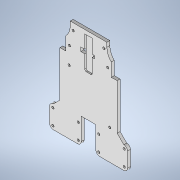
# Autodesk Inventor part: Основа робота
Saved by Autodesk Inventor 2020 (Build 240168000, 168)
## iProperties
Created: 2021-02-28
Part Number: Основа робота
Material: Типовые
Document SubType Name: Обычные детали
Designer: Антон
Density: 1 g/cm^3
Appearance: По умолчанию
Mass: 52.0111 g
Surface Area: 352.197 cm^2
Volume: 52.0111 cm^3
Sheet Metal Rule: По умолчанию
Author: Антон
Autodesk Inventor part; units mm, degrees
ref_plane "YZ Plane" through (0, 0, 0) normal (1, 0, 0) x (0, 1, 0)
ref_plane "XZ Plane" through (0, 0, 0) normal (0, 1, 0) x (-1, 0, 0)
ref_plane "XY Plane" through (0, 0, 0) normal (0, 0, 1) x (1, 0, 0)
sketch "Эскиз1" plane through (0, 0, 0) normal (0, 0, 1) x (1, 0, 0)
  line L0 (0, 0) -> (39, 0)
  line L1 (39, 0) -> (39, 139.6)
  line L2 (39, 139.6) -> (0, 139.6)
  line L3 (0, 139.6) -> (0, 0)
  line L4 (0, 0) -> (-14.05, 0)
  line L5 (-14.05, 0) -> (-14.05, 30.3)
  line L6 (-14.05, 30.3) -> (0, 30.3)
  line L7 (0, 30.3) -> (0, 0)
  line L8 (-14.05, 0) -> (-9.5, 0)
  line L9 (-9.5, 0) -> (-9.5, 4.55)
  line L10 (-9.5, 4.55) -> (-9.5, 25.75)
  circle A0 centre (-9.5, 25.75) radius 1.6
  circle A1 centre (-9.5, 4.55) radius 1.6
  line L11 (39, 0) -> (29, 0)
  line L12 (29, 0) -> (29, 35)
  line L13 (29, 35) -> (39, 35)
  line L14 (39, 35) -> (39, 0)
  line L15 (29, 4.55) -> (25, 4.55)
  line L16 (29, 25.75) -> (25, 25.75)
  circle A2 centre (25, 25.75) radius 1.6
  circle A3 centre (25, 4.55) radius 1.6
  line L17 (39, 139.6) -> (39, 130.4)
  line L18 (39, 130.4) -> (18, 130.4)
  circle A4 centre (18, 130.4) radius 1.6
  line L19 (39, 139.6) -> (34, 139.6)
  line L20 (34, 139.6) -> (18, 139.6)
  line L21 (25, 25.75) -> (25, 4.55)
  circle A5 centre (12.95, 110.25) radius 1.6
  line L22 (0, 139.6) -> (14, 139.6)
  line L23 (14, 139.6) -> (14, 119.25)
  line L24 (14, 119.25) -> (0, 119.25)
  line L25 (0, 119.25) -> (0, 139.6)
  line L26 (0, 119.25) -> (8, 119.25)
  line L27 (8, 119.25) -> (8, 101.25)
  line L28 (8, 101.25) -> (0, 101.25)
  line L29 (0, 101.25) -> (0, 119.25)
  point P0 (0, 30.3)
  point P1 (29, 0)
  point P2 (39, 35)
  point P3 (0, 182.1)
  point P4 (25, 15.15)
  point P5 (-9.5, 15.15)
  point P6 (0, 119.25)
  point P7 (8, 119.25)
  point P8 (0, 101.25)
  dimension "d0" = 39
  dimension "d1" = 139.6
  dimension "d191" = 14.05
  dimension "d192" = 30.3
  dimension "d207" = 4.55
  dimension "d208" = 4.55
  dimension "d209" = 21.2
  dimension "d210" = 10
  dimension "d211" = 35
  dimension "d215" = 4
  dimension "d290" = 3.2
  dimension "d309" = 21
  dimension "d311" = 3.2
  dimension "d325" = 9.2
  dimension "d387" = 21.2
  dimension "d418" = 4.55
  dimension "d419" = 12.95
  dimension "d420" = 29.35
  dimension "d421" = 3.2
  dimension "d424" = 14
  dimension "d425" = 20.35
  dimension "d427" = 8
  dimension "d428" = 18
  constraints: 60 end point, 11 parallel, 8 perpendicular, 7 horizontal, 6 centre point, 6 point on line, 5 coincident, 3 equal radius, 2 midpoint, 1 collinear, 1 horizontal alignment, 1 vertical
  measures "d0" distance of L2.end L1.end
  measures "d1" distance of L1.end L0.end
  measures "d191" distance of L5.end L6.end
  measures "d192" distance of L4.end L5.end
  measures "d207" distance of L4.end L8.end
  measures "d208" distance of L8.end L9.end
  measures "d209" distance of L9.end L10.end
  measures "d210" distance of L12.end L13.end
  measures "d211" distance of L11.end L12.end
  measures "d215" distance of L16.start L16.end
  measures "d290" diameter of A2
  measures "d309" distance of L17.end L18.end
  measures "d311" diameter of A4
  measures "d325" distance from line of L19.end L18
  measures "d387" distance of L21.end L21.start
  measures "d418" distance from line of L0 L15.end
  measures "d419" distance from line of L3 A5.centre
  measures "d420" distance from line of L2 A5.centre
  measures "d421" diameter of A5
  measures "d424" distance of L23.end L24.end
  measures "d425" distance of L22.end L23.end
  measures "d427" distance of L27.end L28.end
  measures "d428" distance of L26.end L27.end
extrude "Выдавливание1" add sketch "Эскиз1" along normal blind 4 contours L3 L28 L27 L24 L23 L2 L1 L13 L12 L16 A2 L21 A3 L15 L0 | L4 L5 L6 L3 | L15 A3 L21 A2 L16 L12
mirror "Зеркальное отражение1" about plane through (39, 35, 0) normal (1, 0, 0) of "Выдавливание1"
sketch "Эскиз18" plane through (0, 0, 4) normal (0, 0, 1) x (1, 0, 0)
  line L0 (39, 139.6) -> (39, 86.75)
  line L1 (39, 86.75) -> (12.6, 86.75)
  line L2 (39, 86.75) -> (39, 41.05)
  line L3 (39, 41.05) -> (67.8, 41.05)
  line L4 (14, 139.6) -> (64, 139.6) projected
  point P0 (-4.55, 159.6)
  point P1 (82.55, 159.6)
  point P2 (0, 139.6)
  point P3 (78, 139.6)
  dimension "d218" = 52.85
  dimension "d220" = 26.4
  dimension "d221" = 45.7
  dimension "d222" = 28.8
  constraints: 8 end point, 2 horizontal, 2 vertical, 2 other
  measures "d218" distance of L0.start L0.end
  measures "d220" distance of L0.end L1.end
  measures "d221" distance of L0.end L2.end
  measures "d222" distance of L2.end L3.end
hole "Отверстие10" at (12.6, 86.75, 4) at (67.8, 41.05, 4) direction (0, 0, -1) diameter 3.2 end through all
fillet "Сопряжение2" radius 5.05 6 edges at (-14.05, 30.3, 2) (-14.05, 0, 2) (29, 0, 2) (49, 0, 2) (92.05, 0, 2) (92.05, 30.3, 2)
sketch "Эскиз19" plane through (0, 0, 0) normal (0, 0, -1) x (-1, 0, 0)
  line L0 (-14, 139.6) -> (-64, 139.6) projected
  circle A0 centre (-12.6, 86.75) radius 1.6 projected
  circle A1 centre (-12.6, 86.75) radius 1.6 projected
  line L1 (-15.4, 88.3666) -> (-12.6, 89.9832)
  line L2 (-12.6, 89.9832) -> (-9.8, 88.3666)
  line L3 (-9.8, 88.3666) -> (-9.8, 85.1334)
  line L4 (-9.8, 85.1334) -> (-12.6, 83.5168)
  line L5 (-12.6, 83.5168) -> (-15.4, 85.1334)
  line L6 (-15.4, 85.1334) -> (-15.4, 88.3666)
  line L7 (0, 101.25) -> (0, 30.3) projected
  point P0 (0, 139.6)
  point P1 (-78, 139.6)
  point P2 (0, 119.25)
  dimension "d423" = 5.6
  constraints: 12 end point, 1 coincident, 1 parallel, 13 other
  measures "d423" distance between parallel lines of L3 L6
extrude "Выдавливание7" cut sketch "Эскиз19" against normal blind 2.6 contours A0 | L1 L2 L3 L4 L5 L6
chamfer "Фаска1" distance 9 angle 45 2 edges at (0, 30.3, 2) (78, 30.3, 2)
sketch "Эскиз21" plane through (0, 0, 4) normal (0, 0, 1) x (1, 0, 0)
  line L0 (39, 139.6) -> (39, 134.4)
  line L1 (44.05, 134.4) -> (33.95, 134.4)
  line L2 (33.95, 134.4) -> (33.95, 90.75)
  line L3 (33.95, 90.75) -> (44.05, 90.75)
  line L4 (44.05, 90.75) -> (44.05, 134.4)
  line L5 (42, 92.8) -> (36, 92.8) construction
  line L6 (42, 90.75) -> (36, 90.75)
  line L7 (36, 94.85) -> (42, 94.85)
  arc A0 (42, 90.75) -> (42, 94.85) centre (42, 92.8) ccw
  arc A1 (36, 94.85) -> (36, 90.75) centre (36, 92.8) ccw
  line L8 (14, 139.6) -> (64, 139.6) projected
  point P0 (0, 0)
  point P1 (39, 92.8)
  point P2 (33.95, 92.8)
  point P3 (42, 90.75)
  point P4 (44.05, 92.8)
  point P5 (-4.55, 159.6)
  point P6 (82.55, 159.6)
  point P7 (0, 139.6)
  point P8 (78, 139.6)
  dimension "d297" = 10.1
  dimension "d298" = 43.65
  dimension "d299" = 5.2
  dimension "d307" = 4.1
  constraints: 18 end point, 6 tangent, 4 point on circle, 3 parallel, 2 centre point, 2 midpoint, 2 perpendicular, 1 collinear, 1 horizontal, 1 vertical, 2 other
  measures "d297" distance of L3.end L2.end
  measures "d298" distance of L2.end L1.end
  measures "d299" distance of L0.start L0.end
  measures "d307" distance between parallel lines of L3 L7
extrude "Выдавливание9" cut sketch "Эскиз21" against normal blind 2 contours L4 A0 L7 A1 L2 L1 | A0 L3 A1 L7
sketch "Эскиз25" plane through (0, 0, 0) normal (0, 0, -1) x (-1, 0, 0)
  circle A0 centre (-25, 25.75) radius 1.6 projected
  circle A1 centre (-25, 4.55) radius 1.6 projected
  circle A2 centre (9.5, 25.75) radius 1.6 projected
  circle A3 centre (9.5, 4.55) radius 1.6 projected
  circle A4 centre (-53, 25.75) radius 1.6 projected
  circle A5 centre (-53, 4.55) radius 1.6 projected
  circle A6 centre (-87.5, 4.55) radius 1.6 projected
  circle A7 centre (-87.5, 25.75) radius 1.6 projected
  circle A8 centre (-67.8, 41.05) radius 1.6 projected
  circle A9 centre (-12.6, 86.75) radius 1.6 projected
  circle A10 centre (-18, 130.4) radius 1.6 projected
  circle A11 centre (-60, 130.4) radius 1.6 projected
  circle A12 centre (-65.05, 110.25) radius 1.6 projected
  circle A13 centre (-12.95, 110.25) radius 1.6 projected
  circle A14 centre (-65.05, 110.25) radius 1.6 projected
  circle A15 centre (-12.95, 110.25) radius 1.6 projected
  point P0 (0, 0)
  constraints: 14 coincident
pattern_sketch "Массив по эскизу1" of "Выдавливание7" from (12.6, 86.75, 0) copies at (25, 25.75, 0) at (25, 4.55, 0) at (-9.5, 25.75, 0) at (-9.5, 4.55, 0) at (53, 25.75, 0) at (53, 4.55, 0) at (87.5, 4.55, 0) at (87.5, 25.75, 0) at (67.8, 41.05, 0) at (18, 130.4, 0) at (60, 130.4, 0) at (65.05, 110.25, 0) at (12.95, 110.25, 0)
sketch "Эскиз29" plane through (0, 0, 4) normal (0, 0, 1) x (1, 0, 0)
  line L0 (47.05, 111.6) -> (44.05, 111.6)
  line L1 (44.05, 111.6) -> (44.05, 115.6)
  line L2 (44.05, 115.6) -> (47.05, 115.6)
  line L3 (47.05, 115.6) -> (47.05, 111.6)
  line L4 (44.05, 134.4) -> (44.05, 92.8) projected
  line L5 (33.95, 110.85) -> (28.45, 110.85)
  line L6 (28.45, 110.85) -> (28.45, 116.35)
  line L7 (28.45, 116.35) -> (33.95, 116.35)
  line L8 (33.95, 116.35) -> (33.95, 110.85)
  line L9 (33.95, 92.8) -> (33.95, 134.4) projected
  point P0 (0, 0)
  point P1 (44.05, 113.6)
  point P2 (44.05, 136.615)
  point P3 (33.95, 113.6)
  point P4 (33.95, 136.615)
  dimension "d405" = 3
  dimension "d406" = 4
  dimension "d407" = 5.5
  dimension "d408" = 5.5
  constraints: 16 end point, 4 midpoint, 4 parallel, 2 horizontal, 2 perpendicular
  measures "d405" distance of L1.end L2.end
  measures "d406" distance of L0.end L1.end
  measures "d407" distance of L5.start L5.end
  measures "d408" distance of L5.end L6.end
extrude "Выдавливание13" cut sketch "Эскиз29" against normal through all
fillet "Сопряжение10" radius 20.35 2 edges at (64, 119.25, 2) (14, 119.25, 2)
equation "\"Радиус_гибки\" = Толщина"
equation "\"Ширина_просечки\" = Толщина"
equation "\"Глубина_просечки\" = 0.5 * Толщина"
equation "\"Размер_просечки\" = 4 * Толщина"
equation "\"Мин_остаток\" = 2 * Толщина"
equation "\"Радиус_перехода\" = Радиус_гибки"
equation "\"Радиус_Якоби\" = Толщина"
equation "\"Размер_зазора\" = Толщина"
equation "\"Гайка_М3_з\" = 5.6"
equation "\"d130\" = 5.6"
equation "\"Толщина\" = 0.5"
